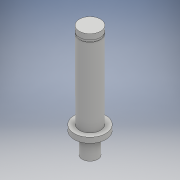
# Autodesk Inventor part: tige_roue
Saved by Autodesk Inventor 2018 (Build 220112000, 112)
## iProperties
Created: 2019-11-06
Part Number: tige_roue
Material: Generic
Document SubType Name: Modeling
Designer: hugo
Density: 1 g/cm^3
Appearance: Default
Author: hugo
Autodesk Inventor part; units mm, degrees
ref_plane "YZ Plane" through (0, 0, 0) normal (1, 0, 0) x (0, 1, 0)
ref_plane "XZ Plane" through (0, 0, 0) normal (0, 1, 0) x (-1, 0, 0)
ref_plane "XY Plane" through (0, 0, 0) normal (0, 0, 1) x (1, 0, 0)
sketch "Sketch1" plane through (0, 0, 0) normal (1, 0, 0) x (0, 1, 0)
  line L0 (0, 0) -> (4, 0)
  line L1 (4, 0) -> (4, -2)
  line L2 (4, -2) -> (3.8, -2)
  line L3 (3.8, -2) -> (3.8, -2.8)
  line L4 (3.8, -2.8) -> (4, -2.8)
  line L5 (4, -2.8) -> (4, -32.6)
  line L6 (4, -32.6) -> (6, -32.6)
  line L7 (6, -32.6) -> (6, -34.6)
  line L8 (6, -34.6) -> (4, -34.6)
  line L9 (3.0077, -42.6) -> (0.0411, -42.6029)
  line L10 (0.0411, -42.6029) -> (0, 0)
  line L11 (4, -34.6) -> (3, -34.6)
  line L12 (3, -34.6) -> (3.0077, -42.6)
  dimension "d0" = 4
  dimension "d1" = 2
  dimension "d2" = 0.2
  dimension "d3" = 0.8
  dimension "d4" = 29.8
  dimension "d5" = 2
  dimension "d6" = 2
  dimension "d9" = 1
  dimension "d10" = 8
  constraints: 26 end point, 6 horizontal, 5 perpendicular, 1 vertical
  measures "d0" distance of L0.start L0.end
  measures "d1" distance of L0.end L1.end
  measures "d2" distance of L1.end L2.end
  measures "d3" distance of L2.end L3.end
  measures "d4" distance of L4.end L5.end
  measures "d5" distance of L5.end L6.end
  measures "d6" distance of L6.end L7.end
  measures "d9" distance of L8.end L11.end
  measures "d10" distance of L11.end L9.start
revolve "Revolution1" add sketch "Sketch1" angle 360 about axis through (0, 0.0411, -42.6029) along (0, -0.0009653, 0.9999995)
equation "\"d10\" = lr"
equation "\"lr\" = 8"
body "Solid1"
